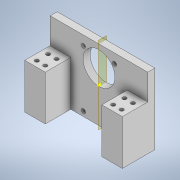
# Autodesk Inventor part: Front_plate
Saved by Autodesk Inventor 2022 (Build 260153000, 153)
## iProperties
Created: 2021-07-29
Part Number: Front_plate
Material: Generic
Document SubType Name: Modeling
Designer: exllu
Density: 1 g/cm^3
Appearance: Default
Author: exllu
Autodesk Inventor part; units mm, degrees
ref_plane "YZ Plane" through (0, 0, 0) normal (1, 0, 0) x (0, 1, 0)
ref_plane "XZ Plane" through (0, 0, 0) normal (0, 1, 0) x (-1, 0, 0)
ref_plane "XY Plane" through (0, 0, 0) normal (0, 0, 1) x (1, 0, 0)
sketch "Sketch1" plane through (0, 0, 0) normal (0, 0, 1) x (1, 0, 0)
  line L0 (0, 0) -> (36, 0)
  line L1 (36, 0) -> (36, 25)
  line L2 (36, 25) -> (-36, 25)
  line L3 (-36, 25) -> (-36, -25)
  line L4 (-36, -25) -> (36, -25)
  line L5 (36, -25) -> (36, 25)
  dimension "d0" = 36
  dimension "d1" = 25
  dimension "d2" = 72
  dimension "d3" = 50
  constraints: 12 end point, 2 horizontal, 2 parallel, 1 perpendicular, 1 vertical
  measures "d0" distance of L0.start L0.end
  measures "d1" distance of L0.end L1.end
  measures "d2" distance of L4.end L3.end
  measures "d3" distance of L3.end L2.end
extrude "Extrusion1" add sketch "Sketch1" along normal blind 5
sketch "Sketch2" plane through (0, 0, 5) normal (0, 0, 1) x (1, 0, 0)
  line L0 (0, 0) -> (0, -25)
  line L1 (-36, -25) -> (36, -25) projected
  line L2 (0, -25) -> (0, 10.25)
  circle A0 centre (0, 10.25) radius 11.25
  dimension "d6" = 35.25
  dimension "d7" = 22.5
  constraints: 4 end point, 1 centre point, 1 coincident, 1 midpoint, 1 point on line
  measures "d6" distance of L0.end L2.end
  measures "d7" diameter of A0
extrude "Extrusion2" cut sketch "Sketch2" against normal blind 22.5
sketch "Sketch3" plane through (0, 0, 5) normal (0, 0, 1) x (1, 0, 0)
  line L0 (0, 0) -> (11, 0)
  line L1 (11, -24.8696) -> (11, -21.6196)
  circle A0 centre (11, -21.6196) radius 1.475
  line L2 (0, 0) -> (0, -3.6992)
  circle A1 centre (-11, -21.6196) radius 1.475
  line L3 (11, -21.6196) -> (11, 18.3804)
  line L4 (11, -21.6196) -> (11, -1.6196)
  line L5 (11, -1.6196) -> (-3.4092, -1.6196)
  circle A2 centre (11, 18.3804) radius 1.475
  circle A3 centre (-11, 18.3804) radius 1.475
  point P0 (0, -1.6196)
  point P1 (11, -20.1446)
  point P2 (11, -23.0946)
  dimension "d10" = 11
  dimension "d11" = 3.25
  dimension "d12" = 2.95
  dimension "d15" = 40
  dimension "d16" = 20
  constraints: 12 end point, 4 centre point, 3 symmetric about line, 2 vertical, 1 coincident, 1 horizontal, 1 midpoint, 1 perpendicular, 3 other
  measures "d10" distance of L0.start L0.end
  measures "d11" distance of L1.start L1.end
  measures "d12" diameter of A0
  measures "d15" distance of L3.start L3.end
  measures "d16" distance of L3.start L4.end
extrude "Extrusion3" cut sketch "Sketch3" against normal blind 5 contours A0 L1 L3 | L3 L1 A0 | A1
sketch "Sketch4" plane through (0, 0, 5) normal (0, 0, 1) x (1, 0, 0)
  point P0 (0, 0)
extrude "Extrusion4" cut sketch "Sketch3" against normal blind 5 contours A2 | A3
sketch "Sketch5" plane through (36, -25, 0) normal (1, 0, 0) x (0, 0, -1)
  line L0 (0, 0) -> (0, 50) projected
  line L1 (-5, 0) -> (-5, 50) projected
  line L2 (0, 0) -> (-5, 0)
  line L3 (-5, 0) -> (-5, 50)
  line L4 (-5, 50) -> (0, 50)
  line L5 (0, 50) -> (0, 0)
  point P0 (0, 25)
  dimension "d19" = 5
  constraints: 8 end point, 2 parallel, 1 horizontal, 1 perpendicular
  measures "d19" distance of L1.end L4.end
ref_plane "Work Plane1" through (0, -25, 0) normal (1, 0, 0) x (0, 0, -1)
extrude "Extrusion5" cut sketch "Sketch5" against normal blind 1.5
mirror "Mirror1" about plane through (0, -25, 0) normal (1, 0, 0) of "Extrusion5"
sketch "Sketch6" plane through (34.5, -25, 0) normal (1, 0, 0) x (0, 0, -1)
  line L0 (-5, 0) -> (0, 0) projected
  line L1 (-5, 0) -> (-23, 0)
  line L2 (-23, 0) -> (-23, 34.75)
  line L3 (-23, 34.75) -> (-5, 34.75)
  line L4 (-5, 50) -> (-5, 0) projected
  line L5 (-5, 34.75) -> (-5, 0)
  point P0 (0, 25)
  dimension "d22" = 18
  dimension "d23" = 34.75
  dimension "d24" = 18
  constraints: 8 end point, 2 horizontal, 1 perpendicular
  measures "d22" distance of L0.start L1.end
  measures "d23" distance of L1.end L2.end
  measures "d24" distance of L2.end L3.end
extrude "Extrusion6" add sketch "Sketch6" against normal blind 14.5
mirror "Mirror2" about plane through (0, -25, 0) normal (1, 0, 0) of "Extrusion6"
sketch "Sketch7" plane through (34.5, 9.75, 23) normal (0, 1, 0) x (1, 0, 0)
  line L0 (0, 0) -> (-14.5, 0) projected
  line L1 (0, 18) -> (0, 23) projected
  line L2 (0, 0) -> (0, 18)
  line L3 (0, 18) -> (0, 4)
  line L4 (0, 23) -> (0, 0) projected
  point P0 (-34.5, 23)
  point P1 (-10.5, 4)
  point P2 (-4.5, 4)
  constraints: 4 end point, 1 point on line, 1 vertical
hole "Hole1" at (24, 9.75, 19) at (30, 9.75, 19) direction (0, -1, 0) diameter 2.7 depth 28 tip angle 118
mirror "Mirror3" about plane through (0, -25, 0) normal (1, 0, 0) of "Hole1"
sketch "Sketch8" plane through (34.5, 9.75, 23) normal (0, 1, 0) x (1, 0, 0)
  line L0 (0, 23) -> (0, 0) projected
  line L1 (0, 0) -> (0, 4)
  line L2 (0, 4) -> (-4.5, 4)
  line L3 (-4.5, 4) -> (-4.5, 12)
  line L4 (-4.5, 12) -> (-10.5, 12)
  point P0 (-34.5, 23)
  dimension "d45" = 4
  dimension "d46" = 4.5
  dimension "d47" = 8
  dimension "d48" = 6
  constraints: 8 end point, 2 coincident, 2 perpendicular, 1 horizontal, 1 point on line
  measures "d45" distance of L0.end L1.end
  measures "d46" distance of L1.end L2.end
  measures "d47" distance of L2.end L3.end
  measures "d48" distance of L3.end L4.end
hole "Hole2" at (24, 9.75, 11) at (30, 9.75, 11) direction (0, -1, 0) diameter 2.7 depth 28 tip angle 118
mirror "Mirror4" about plane through (0, -25, 0) normal (1, 0, 0) of "Hole2"
sketch "Sketch9" plane through (-34.5, 9.75, 23) normal (0, 1, 0) x (1, 0, 0)
  line L0 (0, 0) -> (14.5, 0) projected
  line L1 (0, 0) -> (74.2049, 0)
  line L2 (74.2049, 0) -> (74.2049, 18)
  line L3 (74.2049, 18) -> (0, 18)
  line L4 (0, 18) -> (0, 0)
  point P0 (34.5, 23)
  constraints: 8 end point, 2 parallel, 1 horizontal, 1 perpendicular
extrude "Extrusion7" cut sketch "Sketch9" against normal blind 3
ref_plane "Work Plane2" through (0, -25, 0) normal (1, 0, 0) x (0, 0, -1)
equation "\"d8\" = d7"
body "Solid1"
